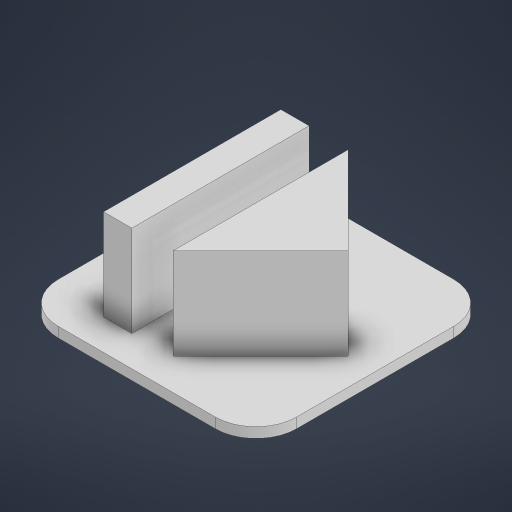
# Autodesk Inventor part: guzik_stop
Saved by Autodesk Inventor 2024.4 (Build 284460000, 460)
## iProperties
Created: 2026-03-18
Part Number: guzik_stop
Material: Ogólny
Document SubType Name: Modeling
Designer: User
Density: 1 g/cm^3
Appearance: Domyślna
Author: User
Autodesk Inventor part; units mm, degrees
ref_plane "YZ Plane" through (0, 0, 0) normal (1, 0, 0) x (0, 1, 0)
ref_plane "XZ Plane" through (0, 0, 0) normal (0, 1, 0) x (-1, 0, 0)
ref_plane "XY Plane" through (0, 0, 0) normal (0, 0, 1) x (1, 0, 0)
sketch "Szkic1" plane through (0, 0, 0) normal (0, 1, 0) x (-1, 0, 0)
  line L0 (5.1235, 4.3458) -> (-4.6765, 4.3458)
  line L1 (-4.6765, 4.3458) -> (-4.6765, -5.4542)
  line L2 (-4.6765, -5.4542) -> (5.1235, -5.4542)
  line L3 (5.1235, -5.4542) -> (5.1235, 4.3458)
  line L4 (5.1235, 4.3458) -> (-4.6765, -5.4542) construction
  line L5 (-4.6765, 4.3458) -> (5.1235, -5.4542) construction
  line L6 (0.2235, -0.5542) -> (2.6735, -0.5542)
  line L7 (3.4085, 3.8558) -> (1.9385, 3.8558)
  line L8 (1.9385, 3.8558) -> (1.9385, -4.9642)
  line L9 (1.9385, -4.9642) -> (3.4085, -4.9642)
  line L10 (3.4085, -4.9642) -> (3.4085, 3.8558)
  line L11 (3.4085, 3.8558) -> (1.9385, -4.9642) construction
  line L12 (1.9385, 3.8558) -> (3.4085, -4.9642) construction
  line L13 (0.2235, -0.5542) -> (0.0314, -0.5542)
  line L14 (0.0314, -0.5542) -> (0.0314, -4.9642)
  line L15 (0.0314, -0.5542) -> (-4.3786, -0.5542)
  line L16 (-4.3786, -0.5542) -> (0.0314, -4.9642)
  line L17 (-4.3786, -0.5542) -> (0.0314, 3.8558)
  line L18 (0.0314, -0.5542) -> (0.0314, 3.8558)
  line L19 (-5.6565, 5.3258) -> (6.1035, 5.3258)
  line L20 (6.1035, 5.3258) -> (6.1035, -6.4342)
  line L21 (6.1035, -6.4342) -> (-5.6565, -6.4342)
  line L22 (-5.6565, -6.4342) -> (-5.6565, 5.3258)
  line L23 (-5.6565, 5.3258) -> (6.1035, -6.4342) construction
  line L24 (6.1035, 5.3258) -> (-5.6565, -6.4342) construction
  point P0 (0, 0)
  dimension "d0" = 9.8
  dimension "d1" = 9.8
  dimension "d2" = 2.45
  dimension "d3" = 1.47
  dimension "d4" = 8.82
  dimension "d5" = 0.1921
  dimension "d6" = 4.41
  dimension "d7" = 4.41
  dimension "d8" = 11.76
  dimension "d9" = 11.76
  constraints: 50 end point, 6 midpoint, 6 parallel, 5 horizontal, 3 perpendicular, 1 point on line, 1 symmetric about line, 1 vertical
  measures "d0" distance of L2.end L1.end
  measures "d1" distance of L1.end L0.end
  measures "d2" distance of L13.start L6.end
  measures "d3" distance of L9.end L9.start
  measures "d4" distance of L9.start L7.end
  measures "d5" distance of L13.start L18.start
  measures "d6" distance of L18.start L16.end
  measures "d7" distance of L18.start L15.end
  measures "d8" distance of L20.end L21.end
  measures "d9" distance of L19.end L20.end
extrude "Wyciągnięcie proste1" add sketch "Szkic1" along normal blind 0.5 contours L3 L2 L1 L0 | L10 L9 L8 L7 | L14 L16 L15 | L15 L17 L18 | L19 L20 L21 L22
extrude "Wyciągnięcie proste2" add sketch "Szkic1" along normal blind 5 contours L10 L9 L8 L7 | L14 L16 L15 | L15 L17 L18
fillet "Zaokrąglenie1" radius 2 4 edges at (5.6565, 0.25, 5.3258) (-6.1035, 0.25, 5.3258) (5.6565, 0.25, -6.4342) (-6.1035, 0.25, -6.4342)
offset faces "Rozmiar1" outward -0.04 faces at (-1.9385, 2, 0.9158) (-2.4285, 2, -4.9642) (-3.4085, 2, -2.0242) (-2.9185, 2, 3.8558) (-0.0314, 2, -2.0242) (1.4386, 2, 2.3858) (2.9086, 2, -2.0242)
